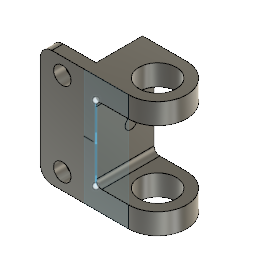
HInge2 (Autodesk Fusion 360 design; units mm, degrees)
Autodesk Fusion 360 part; units mm, degrees
note: some values were not read from the file. Set by a fixed rule: which sketch regions a step uses.
sketch "Sketch1" plane through (0, 0, 0) normal (0, 0, 1) x (1, 0, 0)
  line L0 (0, 0) -> (38, 0)
  line L1 (38, 0) -> (38, 50)
  line L2 (38, 50) -> (0, 50)
  line L3 (0, 50) -> (0, 0)
  circle A0 centre (38, 25) radius 25
  circle A1 centre (38, 25) radius 16
  dimension "d1" = 38
  dimension "d2" = 50
  dimension "d3" = 50
  dimension "d5" = 32
  constraint coincident L0.start L3.end
  constraint horizontal L0
  constraint perpendicular L0 L1
  constraint perpendicular L1 L2
  constraint perpendicular L0 L3
  constraint midpoint L1 A0.centre
  constraint concentric A0 A1
  measures "d1" distance of L0.start L0.end
  measures "d2" distance of L0.end L1.end
  measures "d3" diameter of A0
  measures "d5" diameter of A1
extrude "Extrude1" add sketch "Sketch1" against normal blind 100 contours L0 L2 L3 A0 | L1 A0 A1 | L1 A0 A1
sketch "Sketch2" plane through (0, 0, 0) normal (0, -1, 0) x (1, 0, 0)
  line L0 (38, 0) -> (0, 0)
  line L1 (0, 0) -> (0, -100) construction
  line L2 (0, -100) -> (38, -100)
  line L3 (38, -100) -> (38, 0)
  line L4 (0, -50) -> (10, -50) construction
  line L5 (10, -50) -> (10, -18)
  line L6 (10, -50) -> (10, -82)
  dimension "d8" = 32
  dimension "d9" = 32
  constraint midpoint L1 L4.start
  constraint perpendicular L1 L4
  constraint perpendicular L4 L5
  constraint perpendicular L4 L6
  measures "d8" distance of L4.end L5.end
  measures "d9" distance of L4.end L6.end
sketch "Sketch3" plane through (0, 0, 0) normal (0, -1, 0) x (1, 0, 0)
  line L0 (38, 0) -> (0, 0)
  line L1 (0, 0) -> (0, -100)
  line L2 (0, -100) -> (38, -100)
  line L3 (38, -100) -> (38, 0)
ref_plane "WorkPlane1" through (31.5, 25, -50) normal (0, 0, -1) x (-1, 0, 0)
sketch "Sketch4" plane through (31.5, 25, -50) normal (0, 0, -1) x (1, 0, 0)
sketch "Sketch5" plane through (0, 0, 0) normal (0, 0, 1) x (-1, 0, 0)
  circle A0 centre (-38, -25) radius 16
  arc A1 (-38, 0) -> (-38, -50) centre (-38, -25) ccw
  line L0 (-38, -50) -> (0, -50)
  line L1 (0, -50) -> (0, 0)
  line L2 (0, 0) -> (-38, 0)
  line L3 (0, 0) -> (38, 0)
  line L4 (38, 0) -> (38, -10)
  line L5 (38, -10) -> (0, -10)
  line L6 (0, -10) -> (0, 0)
  dimension "d10" = 38
  dimension "d11" = 10
  constraint coincident L1.end L2.start
  constraint perpendicular L1 L3
  constraint perpendicular L3 L4
  constraint coincident L1 L5.end
  constraint perpendicular L1 L5
  measures "d10" distance of L1.end L3.end
  measures "d11" distance of L3.end L4.end
extrude "Extrude2" add sketch "Sketch5" against normal blind 100 contours L1 L3 L4 L5 L6
sketch "Sketch6" plane through (0, 10, 0) normal (0, 1, 0) x (-1, 0, 0)
  line L0 (38, 0) -> (0, 0)
  line L1 (0, 0) -> (0, -100)
  line L2 (0, -100) -> (38, -100)
  line L3 (38, -100) -> (38, 0)
  line L4 (19, 0) -> (19, -86) construction
  circle A0 centre (19, -86) radius 7.5
  line L5 (19, 0) -> (33, 0) construction
  line L6 (33, 0) -> (33, -14) construction
  line L7 (33, -14) -> (19, -14) construction
  circle A1 centre (19, -14) radius 7.5
  dimension "d14" = 86
  dimension "d15" = 15
  dimension "d16" = 14
  dimension "d17" = 14
  dimension "d18" = 15
  constraint midpoint L0 L4.start
  constraint perpendicular L2 L4
  constraint coincident L4.end A0.centre
  constraint perpendicular L4 L5
  constraint perpendicular L0 L6
  constraint coincident L4 L7.end
  constraint perpendicular L4 L7
  constraint coincident L7.end A1.centre
  measures "d14" distance of L4.start L4.end
  measures "d15" diameter of A0
  measures "d16" distance of L4.start L5.end
  measures "d17" distance of L5.end L6.end
  measures "d18" diameter of A1
extrude "Extrude3" cut sketch "Sketch6" against normal blind 10 contours A0 | A1
fillet "Fillet1" radius 10 1 edges at (-38, 5, 0)
fillet "Fillet2" radius 10 1 edges at (-38, 5, -100)
ref_plane "WorkPlane2" through (17.5, 25, -50) normal (0, 0, 1) x (1, 0, 0)
sketch "Sketch7" plane through (17.5, 25, -50) normal (0, 0, 1) x (1, 0, 0)
  line L0 (-17.4789, 13.5699) -> (-7.4789, 13.5699) construction
  line L1 (-7.4789, 25.0534) -> (-7.4789, -25)
  line L2 (-7.4789, 25.0534) -> (50, 25.0534)
  line L3 (50, 25.0534) -> (50, -25)
  line L4 (50, -25) -> (-7.4789, -25)
  dimension "d25" = 10
  constraint horizontal L0
  constraint perpendicular L0 L1
  constraint perpendicular L1 L2
  constraint perpendicular L2 L3
  constraint perpendicular L1 L4
  measures "d25" distance of L0.start L0.end
extrude "Extrude4" cut sketch "Sketch7" along normal mid plane 64
sketch "Sketch8" plane through (0, 0, 0) normal (-1, 0, 0) x (0, -1, 0)
  line L0 (-10, -100) -> (-10, 0)
  line L1 (-10, 0) -> (-50, 0)
  line L2 (-50, 0) -> (-50, -100)
  line L3 (-50, -100) -> (-10, -100)
  line L4 (-50, -50) -> (-10, -50) construction
  circle A0 centre (-30, -50) radius 5
  dimension "d28" = 10
  constraint midpoint L2 L4.start
  constraint midpoint L0 L4.end
  constraint midpoint L4 A0.centre
  measures "d28" diameter of A0
fillet "Fillet3" radius 5 1 edges at (10.0211, 25, -18)
fillet "Fillet4" radius 5 1 edges at (10.0211, 25, -82)
extrude "Extrude5" cut sketch "Sketch8" against normal blind 10 contours A0
